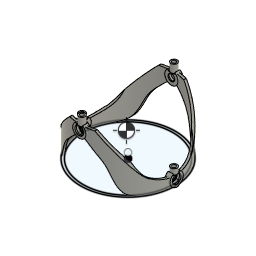
Thrust_Puck (Autodesk Fusion 360 design; units mm, degrees)
Autodesk Fusion 360 part; units mm, degrees
sketch "Sketch1" plane through (0, 0, 0) normal (0, 0, 1) x (1, 0, 0)
  circle A0 centre (0, 0) radius 85
  circle A1 centre (0, 0) radius 89.5
  dimension "d1" = 170
  dimension "d2" = 179
  constraint coincident A0.centre A1.centre
  measures "d1" diameter of A0
  measures "d2" diameter of A1
extrude "Extrude1" add sketch "Sketch1" along normal blind 100 makes body 1
sketch "Sketch2" plane through (0, 0, 0) normal (0, 1, 0) x (1, 0, 0)
  spline S0 degree 5 poles (-82.6314, 0.4087) (-82.0074, 0.4087) (-80.7085, 0.3877) (-78.6073, 0.2932) (-75.5399, 0.027) (-71.4891, -0.6158) (-67.4993, -1.6561) (-63.8301, -3.1648) (-60.6407, -5.162) (-57.9471, -7.6019) (-55.6798, -10.404) (-53.7216, -13.476) (-51.9509, -16.7379) (-50.2883, -20.1498) (-48.6906, -23.7016) (-47.1334, -27.3941) (-45.598, -31.2234) (-44.0565, -35.164) (-42.4581, -39.1526) (-40.7392, -43.1077) (-38.8336, -46.9492) (-36.6835, -50.6191) (-34.2493, -54.0995) (-31.5216, -57.4381) (-28.5189, -60.7244) (-25.2807, -64.0516) (-21.8627, -67.4819) (-18.3305, -71.0131) (-14.7549, -74.5386) (-11.2062, -77.824) (-7.749, -80.5776) (-5.0991, -82.1234) (-3.1933, -82.8124) (-1.9608, -83.0498) (-1.3542, -83.113) knots 0 0 0 0 0 0 0.033333 0.066667 0.1 0.133333 0.166667 0.2 0.233333 0.266667 0.3 0.333333 0.366667 0.4 0.433333 0.466667 0.5 0.533333 0.566667 0.6 0.633333 0.666667 0.7 0.733333 0.766667 0.8 0.833333 0.866667 0.9 0.933333 0.966667 1 1 1 1 1 1
  line L0 (0, 50) -> (0, -150)
  spline S1 degree 5 poles (82.6314, 0.4087) (82.0074, 0.4087) (80.7085, 0.3877) (78.6073, 0.2932) (75.5399, 0.027) (71.4891, -0.6158) (67.4993, -1.6561) (63.8301, -3.1648) (60.6407, -5.162) (57.9471, -7.6019) (55.6798, -10.404) (53.7216, -13.476) (51.9509, -16.7379) (50.2883, -20.1498) (48.6906, -23.7016) (47.1334, -27.3941) (45.598, -31.2234) (44.0565, -35.164) (42.4581, -39.1526) (40.7392, -43.1077) (38.8336, -46.9492) (36.6835, -50.6191) (34.2493, -54.0995) (31.5216, -57.4381) (28.5189, -60.7244) (25.2807, -64.0516) (21.8627, -67.4819) (18.3305, -71.0131) (14.7549, -74.5386) (11.2062, -77.824) (7.749, -80.5776) (5.0991, -82.1234) (3.1933, -82.8124) (1.9608, -83.0498) (1.3542, -83.113) knots 0 0 0 0 0 0 0.033333 0.066667 0.1 0.133333 0.166667 0.2 0.233333 0.266667 0.3 0.333333 0.366667 0.4 0.433333 0.466667 0.5 0.533333 0.566667 0.6 0.633333 0.666667 0.7 0.733333 0.766667 0.8 0.833333 0.866667 0.9 0.933333 0.966667 1 1 1 1 1 1
  line L1 (-92.1972, 0.4087) -> (-73.0656, 0.4087)
  line L2 (-9.3525, -82.2794) -> (6.6442, -83.9466)
  line L3 (92.1972, 0.4087) -> (73.0656, 0.4087)
  line L4 (9.3525, -82.2794) -> (-6.6442, -83.9466)
  line L5 (-1.3542, -83.113) -> (1.3542, -83.113)
  line L6 (82.6314, 0.4087) -> (-82.6314, 0.4087)
  line L7 (-82.6314, 0.4087) -> (0, -83.113)
  line L8 (0, -83.113) -> (82.6314, 0.4087)
  point P0 (-64.9736, -2.7923)
  point P1 (-53.4486, -14.0721)
  point P2 (-45.6018, -31.2369)
  point P3 (-36.0722, -51.3984)
  point P4 (-18.8678, -70.4668)
  point P5 (64.9736, -2.7923)
  point P6 (53.4486, -14.0721)
  point P7 (45.6018, -31.2369)
  point P8 (36.0722, -51.3984)
  point P9 (18.8678, -70.4668)
  constraint midpoint S0.start L1
  constraint midpoint S0.end L2
  constraint symmetric S0.start L0 S1.start
  constraint symmetric P0 L0 P5
  constraint symmetric P1 L0 P6
  constraint symmetric P2 L0 P7
  constraint symmetric P3 L0 P8
  constraint symmetric P4 L0 P9
  constraint symmetric S0.end L0 S1.end
  constraint symmetric L0 L1.start L3.start
  constraint symmetric L0 L1.end L3.end
  constraint symmetric L0 L2.start L4.start
  constraint symmetric L0 L2.end L4.end
  constraint coincident L1.end L6
  constraint midpoint L5 L7.end
extrude "Extrude2" cut sketch "Sketch2" along normal mid plane 200 contours S0 L0 L1 L6 L7 | S0 L5 L7 | S1 L5 L8 | L0 S1 L3 L6 L8 bodies 1
sketch "Sketch3" plane through (0, 0, 0) normal (1, 0, 0) x (0, 1, 0)
  spline S0 degree 5 poles (83.9468, 100.2931) (83.6453, 100.3935) (83.0189, 100.5205) (82.0087, 100.49) (80.5209, 100.0069) (78.4407, 98.6841) (76.1925, 96.7152) (73.8622, 94.2198) (71.5469, 91.3261) (69.3385, 88.1448) (67.3019, 84.7303) (65.466, 81.0746) (63.8295, 77.1397) (62.3628, 72.8809) (61.0117, 68.2725) (59.6989, 63.335) (58.3279, 58.1563) (56.7936, 52.8693) (54.9924, 47.6331) (52.8324, 42.6132) (50.2445, 37.9618) (47.1914, 33.8001) (43.6817, 30.1938) (39.7679, 27.1524) (35.5303, 24.6464) (31.0663, 22.6192) (26.4767, 21.0017) (21.8546, 19.7237) (17.2705, 18.7296) (12.7696, 17.9824) (8.3787, 17.4589) (4.964, 17.2089) (2.4599, 17.1142) (0.8158, 17.0923) (0, 17.0916) knots 0 0 0 0 0 0 0.033333 0.066667 0.1 0.133333 0.166667 0.2 0.233333 0.266667 0.3 0.333333 0.366667 0.4 0.433333 0.466667 0.5 0.533333 0.566667 0.6 0.633333 0.666667 0.7 0.733333 0.766667 0.8 0.833333 0.866667 0.9 0.933333 0.966667 1 1 1 1 1 1
  line L0 (0, -50) -> (0, 150)
  spline S1 degree 5 poles (-83.9468, 100.2931) (-83.6453, 100.3935) (-83.0189, 100.5205) (-82.0087, 100.49) (-80.5209, 100.0069) (-78.4407, 98.6841) (-76.1925, 96.7152) (-73.8622, 94.2198) (-71.5469, 91.3261) (-69.3385, 88.1448) (-67.3019, 84.7303) (-65.466, 81.0746) (-63.8295, 77.1397) (-62.3628, 72.8809) (-61.0117, 68.2725) (-59.6989, 63.335) (-58.3279, 58.1563) (-56.7936, 52.8693) (-54.9924, 47.6331) (-52.8324, 42.6132) (-50.2445, 37.9618) (-47.1914, 33.8001) (-43.6817, 30.1938) (-39.7679, 27.1524) (-35.5303, 24.6464) (-31.0663, 22.6192) (-26.4767, 21.0017) (-21.8546, 19.7237) (-17.2705, 18.7296) (-12.7696, 17.9824) (-8.3787, 17.4589) (-4.964, 17.2089) (-2.4599, 17.1142) (-0.8158, 17.0923) (0, 17.0916) knots 0 0 0 0 0 0 0.033333 0.066667 0.1 0.133333 0.166667 0.2 0.233333 0.266667 0.3 0.333333 0.366667 0.4 0.433333 0.466667 0.5 0.533333 0.566667 0.6 0.633333 0.666667 0.7 0.733333 0.766667 0.8 0.833333 0.866667 0.9 0.933333 0.966667 1 1 1 1 1 1
  line L1 (95.2179, 96.5414) -> (72.6757, 104.0448)
  line L2 (13.4021, 17.1028) -> (-13.4021, 17.0804)
  line L3 (-95.2179, 96.5414) -> (-72.6757, 104.0448)
  line L4 (-13.4021, 17.1028) -> (13.4021, 17.0804)
  line L5 (83.9468, 100.2931) -> (-83.9468, 100.2931)
  point P0 (79.5965, 99.3474)
  point P1 (70.3285, 89.5119)
  point P2 (61.1857, 68.7734)
  point P3 (48.7792, 36.1086)
  point P4 (24.2926, 20.4372)
  point P5 (-79.5965, 99.3474)
  point P6 (-70.3285, 89.5119)
  point P7 (-61.1857, 68.7734)
  point P8 (-48.7792, 36.1086)
  point P9 (-24.2926, 20.4372)
  constraint midpoint S0.start L1
  constraint midpoint S0.end L2
  constraint symmetric S0.start L0 S1.start
  constraint symmetric P0 L0 P5
  constraint symmetric P1 L0 P6
  constraint symmetric P2 L0 P7
  constraint symmetric P3 L0 P8
  constraint symmetric P4 L0 P9
  constraint symmetric S0.end L0 S1.end
  constraint symmetric L0 L1.start L3.start
  constraint symmetric L0 L1.end L3.end
  constraint symmetric L0 L2.start L4.start
  constraint symmetric L0 L2.end L4.end
extrude "Extrude3" cut sketch "Sketch3" along normal mid plane 200 contours S0 L0 L5 | L0 S1 L5 bodies 1
sketch "Sketch4" plane through (0, 0, 0) normal (0, 1, 0) x (-1, 0, 0)
  circle A0 centre (0.0574, 91.4999) radius 12.5
  line L0 (-0.0725, 97.8588) -> (5.102, 97.9646)
  circle A1 centre (0.0574, 91.4999) radius 8.2
  circle A2 centre (0.0574, 91.4999) radius 6.3603
  line L1 (0.0345, 99.6998) -> (-5.9248, 99.8055)
  line L2 (-0.0725, 97.8588) -> (-5.247, 97.7531)
  line L3 (5.102, 97.9646) -> (6.0705, 97.9844)
  line L4 (0.0345, 99.6998) -> (6.0337, 99.7817)
  line L5 (-5.9788, 102.4459) -> (-5.8709, 97.1652)
  line L6 (-5.247, 97.7531) -> (-5.8826, 97.7401)
  line L7 (5.978, 102.5088) -> (6.0895, 97.0545)
  line L8 (0.0048, 83.3) -> (-9.4295, 83.3606)
  line L9 (0.0048, 83.3) -> (9.4391, 83.2395)
  point P0 (0, 79)
  point P1 (0, 79)
  dimension "d80" = 25
  dimension "d81" = 16.4
  constraint concentric A0 A1
  constraint coincident P1 A0
  constraint concentric A1 A2
  constraint coincident L0.start A2
  constraint coincident L2.end A1
  constraint tangent A2 L2
  constraint coincident L0.end A1
  constraint tangent L0 A2
  constraint coincident L7.start A0
  constraint coincident L7.end A1
  constraint perpendicular L0 L7
  constraint coincident L5.start A0
  constraint coincident L5.end A1
  constraint perpendicular L2 L5
  constraint coincident L6.end L5
  constraint perpendicular L5 L6
  constraint coincident L3.end L7
  constraint perpendicular L3 L7
  constraint coincident L1.start A1
  constraint midpoint L1.end L5
  constraint midpoint L4.end L7
  constraint coincident A1 L8.start
  constraint coincident A0 L8.end
  constraint tangent A1 L8
  constraint coincident A0 L9.end
  constraint tangent A1 L9
  measures "d80" diameter of A0
  measures "d81" diameter of A1
sketch "Sketch5" plane through (0, 0, 0) normal (0, 0, 1) x (1, 0, 0)
  circle A0 centre (87, -0.0091) radius 3.5
  circle A1 centre (87, -0.0091) radius 6
  circle A2 centre (-87, -0.0091) radius 3.5
  circle A3 centre (-87, -0.0091) radius 6
  circle A4 centre (-0.0658, -87) radius 6
  circle A5 centre (-0.0658, -87) radius 3.5
  circle A6 centre (-0.0658, 87) radius 6
  circle A7 centre (-0.0658, 87) radius 3.5
  dimension "d15" = 7
  dimension "d16" = 12
  dimension "d28" = 7
  dimension "d29" = 12
  dimension "d30" = 7
  dimension "d31" = 12
  dimension "d32" = 7
  dimension "d33" = 12
  dimension "d44" = 87
  dimension "d45" = 87
  dimension "d46" = 87
  dimension "d47" = 87
  constraint concentric A0 A1
  constraint concentric A2 A3
  constraint concentric A4 A5
  constraint concentric A6 A7
  measures "d15" diameter of A0
  measures "d16" diameter of A1
  measures "d28" diameter of A2
  measures "d29" diameter of A3
  measures "d30" diameter of A5
  measures "d31" diameter of A4
  measures "d32" diameter of A7
  measures "d33" diameter of A6
  measures "d44" horizontal distance of origin A0.centre
  measures "d45" horizontal distance of A2.centre origin
  measures "d46" vertical distance of A6.centre origin
  measures "d47" vertical distance of origin A4.centre
extrude "Extrude5" add sketch "Sketch5" along normal blind 16 separate body contours A0 | A1 | A2 | A3 makes body 2 at (92.9925, -0.3082, 10.6667) makes body 3 at (-81.0075, -0.3082, 10.6667)
extrude "Extrude6" add sketch "Sketch5" along normal blind 15 from surface at 16 separate body contours A1 | A3 makes body 4 at (92.9702, -0.6065, 26) makes body 5 at (-81.0298, -0.6065, 26)
extrude "Extrude7" cut sketch "Sketch5" along normal blind 20 from surface at 16 contours A0 | A2 bodies 1
extrude "Extrude8" add sketch "Sketch5" along normal blind 10 from surface at 90 separate body contours A4 | A5 | A6 | A7 makes body 6 at (5.9267, -87.2991, 96.6667) makes body 7 at (5.9267, 86.7009, 96.6667)
extrude "Extrude9" add sketch "Sketch5" along normal blind 15 from surface at 100 separate body contours A4 | A6 makes body 8 at (5.9044, -87.5974, 110) makes body 9 at (5.9044, 86.4026, 110)
sketch "Sketch6" plane through (0, 0, 0) normal (1, 0, 0) x (0, 1, 0)
  circle A0 centre (0, 9.8097) radius 1.5
  dimension "d41" = 3
  measures "d41" diameter of A0
sketch "Sketch7" plane through (0, 0, 0) normal (0, 1, 0) x (1, 0, 0)
  spline S0 degree 5 poles (88.7283, -17.4956) (88.2724, -17.7768) (87.3521, -18.401) (85.9457, -19.5225) (84.0165, -21.3976) (81.4991, -24.4129) (78.8481, -28.1272) (76.0233, -32.5202) (72.9746, -37.515) (69.6531, -42.9997) (66.0187, -48.8392) (62.051, -54.8907) (57.7572, -61.0161) (53.1858, -67.098) (48.4289, -73.0443) (43.6062, -78.7739) (38.8525, -84.2047) (34.3054, -89.2427) (30.0916, -93.7689) (26.3157, -97.6309) (23.0425, -100.6224) (20.8478, -102.1339) (19.4431, -102.6869) (18.6136, -102.7863) (18.2255, -102.7686) knots 0 0 0 0 0 0 0.05 0.1 0.15 0.2 0.25 0.3 0.35 0.4 0.45 0.5 0.55 0.6 0.65 0.7 0.75 0.8 0.85 0.9 0.95 1 1 1 1 1 1
  line L0 (88.7283, -17.4956) -> (88.7283, -100.2418)
  line L1 (88.7283, -100.2418) -> (18.2255, -102.7686)
  line L2 (0, 50) -> (0, -150)
  spline S1 degree 5 poles (-88.7283, -17.4956) (-88.2724, -17.7768) (-87.3521, -18.401) (-85.9457, -19.5225) (-84.0165, -21.3976) (-81.4991, -24.4129) (-78.8481, -28.1272) (-76.0233, -32.5202) (-72.9746, -37.515) (-69.6531, -42.9997) (-66.0187, -48.8392) (-62.051, -54.8907) (-57.7572, -61.0161) (-53.1858, -67.098) (-48.4289, -73.0443) (-43.6062, -78.7739) (-38.8525, -84.2047) (-34.3054, -89.2427) (-30.0916, -93.7689) (-26.3157, -97.6309) (-23.0425, -100.6224) (-20.8478, -102.1339) (-19.4431, -102.6869) (-18.6136, -102.7863) (-18.2255, -102.7686) knots 0 0 0 0 0 0 0.05 0.1 0.15 0.2 0.25 0.3 0.35 0.4 0.45 0.5 0.55 0.6 0.65 0.7 0.75 0.8 0.85 0.9 0.95 1 1 1 1 1 1
  line L3 (96.0354, -12.9872) -> (81.4211, -22.004)
  line L4 (23.906, -103.027) -> (12.5451, -102.5103)
  line L5 (-96.0354, -12.9872) -> (-81.4211, -22.004)
  line L6 (-23.906, -103.027) -> (-12.5451, -102.5103)
  line L7 (-88.7283, -100.2418) -> (-18.2255, -102.7686)
  line L8 (-88.7283, -17.4956) -> (-88.7283, -100.2418)
  line L9 (88.7283, -26.4758) -> (80.0688, -26.4758)
  line L10 (-88.7283, -26.4758) -> (-80.0688, -26.4758)
  point P0 (80.0688, -26.4758)
  point P1 (59.2218, -58.8687)
  point P2 (28.4325, -95.431)
  point P3 (-80.0688, -26.4758)
  point P4 (-59.2218, -58.8687)
  point P5 (-28.4325, -95.431)
  constraint vertical L0
  constraint midpoint S0.start L3
  constraint midpoint S0.end L4
  constraint symmetric S0.start L2 S1.start
  constraint symmetric P0 L2 P3
  constraint symmetric P1 L2 P4
  constraint symmetric P2 L2 P5
  constraint symmetric S0.end L2 S1.end
  constraint symmetric L0.end L2 L7.start
  constraint symmetric L2 L3.start L5.start
  constraint symmetric L2 L3.end L5.end
  constraint symmetric L2 L4.start L6.start
  constraint symmetric L2 L4.end L6.end
  constraint coincident L0 L9.start
  constraint coincident P0 L9.end
  constraint perpendicular L0 L9
  constraint coincident L8 L10.start
  constraint coincident P3 L10.end
  constraint perpendicular L8 L10
extrude "Extrude13" cut sketch "Sketch7" along normal mid plane 180 contours S0 L0 L1 L9 | S1 L7 L8 L10 bodies 1
ref_plane "WorkPlane1" through (0, -85, 0) normal (0, 1, 0) x (0, 0, 1)
sketch "Sketch11" plane through (0, 0, 0) normal (1, 0, 0) x (0, 1, 0)
  circle A0 centre (0.0574, 12.4999) radius 8.2
  circle A1 centre (0.0574, 12.4999) radius 12.5
  circle A2 centre (0.0574, 12.4999) radius 6.3603
  line L0 (-0.0725, 18.8588) -> (-5.247, 18.7531)
  line L1 (-0.0725, 18.8588) -> (5.102, 18.9646)
  line L2 (5.978, 23.5088) -> (6.0895, 18.0545)
  line L3 (-5.9788, 23.4459) -> (-5.8709, 18.1652)
  line L4 (-5.247, 18.7531) -> (-5.8826, 18.7401)
  line L5 (5.102, 18.9646) -> (6.0705, 18.9844)
  line L6 (0.0345, 20.6998) -> (-5.9248, 20.8055)
  line L7 (0.0345, 20.6998) -> (6.0337, 20.7817)
  dimension "d65" = 25
  dimension "d66" = 16.4
  constraint concentric A0 A1
  constraint coincident A1 origin
  constraint concentric A0 A2
  constraint coincident A2 L0.start
  constraint coincident A0 L0.end
  constraint tangent A2 L0
  constraint coincident A0 L1.end
  constraint tangent A2 L1
  constraint coincident A1 L2.start
  constraint coincident A0 L2.end
  constraint perpendicular L1 L2
  constraint coincident A1 L3.start
  constraint coincident A0 L3.end
  constraint perpendicular L0 L3
  constraint coincident L3 L4.end
  constraint perpendicular L3 L4
  constraint coincident L2 L5.end
  constraint perpendicular L2 L5
  constraint coincident A0 L6.start
  constraint midpoint L3 L6.end
  constraint midpoint L2 L7.end
  measures "d65" diameter of A1
  measures "d66" diameter of A0
extrude "Extrude16" add sketch "Sketch11" along normal blind 10 from surface at 82 separate body contours A0 A1 L2 L3 | A0 L2 L5 | A0 L3 L4 | A0 L2 L5 L7 | A0 L3 L4 L6 makes body 10
mirror "Mirror4" about plane through (0, 0, 0) normal (1, 0, 0) of "Extrude16" makes body 11
extrude "Extrude17" cut sketch "Sketch11" along normal mid plane 200 contours A2 | A0 L0 L1 | A0 L0 L1 bodies 1 4 2 10 3 5
extrude "Extrude18" add sketch "Sketch11" along normal blind 2 from surface at 82 separate body contours A0 L0 L1 | A0 L0 L1 makes body 12
extrude "Extrude19" add sketch "Sketch11" against normal blind 2 from surface at -82 contours A0 L0 L1 | A0 L0 L1 bodies 3 5 11
extrude "Extrude20" add sketch "Sketch4" along normal blind 10 from surface at 82 separate body contours A0 A1 L7 L9 | A0 L8 L9 | A0 A1 L5 L8 | A1 L3 L4 L7 | A1 L1 L5 L6 makes body 13
mirror "Mirror5" about plane through (0, 0, 0) normal (0, 1, 0) of "Extrude20" makes body 14
extrude "Extrude21" cut sketch "Sketch4" along normal mid plane 200 contours A2 | L0 A1 L2 | L0 A1 L2 bodies 1 6 7
extrude "Extrude22" add sketch "Sketch4" along normal blind 2 from surface at 82 contours L0 A1 L2 | L0 A1 L2 | A1 L3 L7 | A1 L5 L6 bodies 7 13
extrude "Extrude23" add sketch "Sketch4" against normal blind 2 from surface at -82 contours L0 A1 L2 | L0 A1 L2 | A1 L3 L7 | A1 L5 L6 bodies 6 14
